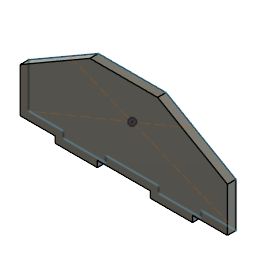
Lateral trasero carga (Autodesk Fusion 360 design; units mm, degrees)
Autodesk Fusion 360 part; units mm, degrees
sketch "Boceto1" plane through (0, 0, 0) normal (0, 0, 1) x (1, 0, 0)
  line L0 (-16, 20) -> (16, 20)
  line L1 (49, 0.9474) -> (49, -20)
  line L2 (-49, -20) -> (-49, 0.9474)
  line L3 (-29.6674, 12.1091) -> (49, -20) construction
  line L4 (29.6674, 12.1091) -> (-49, -20) construction
  line L5 (-49, 0.9474) -> (-16, 20)
  line L6 (16, 20) -> (49, 0.9474)
  line L7 (-12.5, -20) -> (-12.5, -23)
  line L8 (-12.5, -23) -> (-32.5, -23)
  line L9 (-32.5, -23) -> (-32.5, -20)
  line L10 (32.5, -20) -> (32.5, -23)
  line L11 (32.5, -23) -> (12.5, -23)
  line L12 (12.5, -23) -> (12.5, -20)
  line L13 (-32.5, -20) -> (-49, -20)
  line L14 (49, -20) -> (32.5, -20)
  line L15 (12.5, -20) -> (-12.5, -20)
  dimension "d1" = 98
  dimension "d3" = 30
  dimension "d4" = 30
  dimension "d7" = 20
  dimension "d8" = 20
  dimension "d9" = 12.5
  dimension "d10" = 12.5
  dimension "d13" = 33
  dimension "d14" = 16.5
  dimension "d15" = 16.5
  dimension "d16" = 40
  dimension "d17" = 33
  constraint horizontal L0
  constraint perpendicular L0 L1
  constraint parallel L0 L15
  constraint parallel L1 L2
  constraint coincident L3 origin
  constraint coincident L4 origin
  constraint coincident L5 L3.start
  constraint coincident L6 L4.start
  constraint vertical L7
  constraint horizontal L8
  constraint vertical L9
  constraint vertical L10
  constraint horizontal L11
  constraint vertical L12
  constraint collinear L13 L15
  constraint collinear L14 L15
  measures "d1" distance of L1.end L2.start
  measures "d3" angle of L0 L5
  measures "d4" angle of L0 L6
  measures "d7" distance of L7 L9
  measures "d8" distance of L10 L12
  measures "d9" distance of origin L12
  measures "d10" distance of origin L7
  measures "d13" distance of L2 L0.start
  measures "d14" distance of L2 L9
  measures "d15" distance of L1 L10.end
  measures "d16" distance of L0 L13
  measures "d17" distance of L1 L0.end
extrude "Extruir1" add sketch "Boceto1" along normal blind 4
